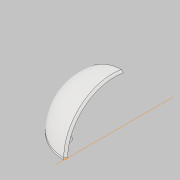
# Autodesk Inventor part: ShellLower
Saved by Autodesk Inventor 2019.2 (Build 232265000, 265)
## iProperties
Created: 2019-01-25
Part Number: ShellLower
Material: ABS-Kunststoff
Document SubType Name: Modeling
Designer: Lion
Density: 1.06 g/cm^3
Appearance: Weiß
Mass: 19.3796 g
Surface Area: 248.39 cm^2
Volume: 18.2826 cm^3
d_inner: 120.000 mm
Author: Lion
## iProperties of the stored document ShellLower_3D-Druck.ipt
Created: 2019-04-11
Part Number: ShellLower_3D-Druck
Material: Generisch
Document SubType Name: Modeling
Designer: Lion
Density: 1 g/cm^3
Appearance: Vorgabe
Author: Lion
Autodesk Inventor part; units mm, degrees
sketch "Skizze1" plane through (0, 0, 0) normal (0, 1, 0) x (-1, 0, 0)
  arc A0 (0, -60) -> (0, 60) centre (0, 0) ccw
  arc A1 (0, -61.5) -> (0, 61.5) centre (0, 0) ccw
  line L0 (0, 60) -> (0, -60) construction
  line L1 (0, 61.5) -> (0, 60)
  line L2 (0, -60) -> (0, -61.5)
  arc A2 (0, 60) -> (0, -60) centre (0, 0) ccw construction
  arc A3 (0, 61.5) -> (0, -61.5) centre (0, 0) ccw construction
  dimension "d_inner" = 120
  dimension "d1" = 123
  constraints: 8 point on circle, 6 end point, 4 centre point, 3 vertical, 2 coincident, 1 midpoint
  measures "d_inner" diameter of A0
  measures "d1" diameter of A1
revolve "Umdrehung1" add sketch "Skizze1" angle 90 about axis through (0, 0, 60) along (0, 0, -1)
sketch "Skizze2" plane through (0, 0, 0) normal (0, -1, 0) x (1, 0, 0)
  arc A0 (0, 60) -> (0, -60) centre (0, 0) ccw projected
  line L0 (0, 60) -> (0, 59)
  line L1 (0, 60) -> (0, -60) construction
  line L2 (-3, 59) -> (-3, 59.925)
  line L3 (0, 59) -> (-3, 59)
  line L4 (0, 0) -> (-60, 0) construction
  dimension "d3" = 1
  dimension "d4" = 3
  constraints: 8 end point, 2 point on circle, 1 horizontal, 1 parallel, 1 perpendicular, 1 point on line
  measures "d3" distance from line of L0.start L3
  measures "d4" distance between parallel lines of L2 L0
sketch "Skizze3" plane through (0, 0, 0) normal (1, 0, 0) x (0, 0, -1)
  line L0 (0, 0) -> (0, 60) construction
  arc A0 (60, 0) -> (-60, 0) centre (0, 0) ccw projected
  line L1 (-60, 0) -> (-59, 0)
  line L2 (-60, 0) -> (60, 0) projected
  line L3 (-59, 0) -> (-59, 2)
  line L4 (-59, 2) -> (-59.9667, 2)
  dimension "d6" = 1
  dimension "d7" = 2
  constraints: 8 end point, 2 point on circle, 2 vertical, 1 perpendicular, 1 point on line
  measures "d6" distance from line of L1.start L3
  measures "d7" distance of L1.end L3.end
ref_plane "Arbeitsebene1" through (0, 0, 0) normal (0, 0, -1) x (-1, 0, 0)
revolve "Umdrehung2" add sketch "Skizze2" angle 180 about axis through (0, 0, 0) along (-1, 0, 0)
revolve "Umdrehung3" add sketch "Skizze3" angle 180 about axis through (0, 0, 0) along (0, -1, 0) contours L4 L3 L1 A0
ref_plane "Arbeitsebene4" through (0, 0, 61) normal (0, 0, -1) x (-1, 0, 0)
chamfer "Fase6" distance 2.5 angle 45 1 edges at (0, 61.5, 0)
sketch "Skizze15" plane through (0, 0, 0) normal (0, -1, 0) x (1, 0, 0)
  line L0 (-2.4995, 61.4492) -> (0, 59) projected
  arc A0 (-2.4995, 61.4492) -> (-2.4995, -61.4492) centre (0, 0) ccw projected
  line L1 (0, -59) -> (-2.4995, -61.4492) projected
  arc A1 (0, 59) -> (0, -59) centre (0, 0) ccw projected
extrude "Extrusion7" add sketch "Skizze15" along normal blind 2.5
chamfer "Fase11" distance 2.5 angle 45 1 edges at (-59, -2.5, 0)
ref_plane "Arbeitsebene21" through (0, 0, 60) normal (0, 1, 0) x (0, 0, -1)
ref_plane "Arbeitsebene20" through (0, 0, 60) normal (1, 0, 0) x (0, 0, -1)
ref_plane "Arbeitsebene25" through (0, 0, 60) normal (0.7071068, 0.7071068, 0) x (0, 0, 1)
ref_plane "Arbeitsebene27" through (-2.4995, -2.5, 61.4492) normal (0, 0, 1) x (1, 0, 0)
ref_plane "Arbeitsebene28" through (-2.4995, -2.5, 2.4492) normal (0, 0, 1) x (1, 0, 0)
ref_plane "Arbeitsebene31" through (-50.9117, 50.9117, 60) normal (0.7071068, -0.7071068, 0) x (0, 0, -1)
ref_plane "Arbeitsebene30" through (-36.7696, 36.7696, 60) normal (0.7071068, -0.7071068, 0) x (0, 0, -1)
ref_plane "Arbeitsebene34" through (-2.4995, 0, -11.4492) normal (0, 0, 1) x (1, 0, 0)
ref_plane "Arbeitsebene33" through (-2.4995, 0, -61.4492) normal (0, 0, 1) x (1, 0, 0)
split "Trennen4" plane through (-2.4995, 0, -11.4492) removes the side toward (0, 0, -1)
ref_plane "Arbeitsebene35" through (0, 0, 60) normal (0.7071068, -0.7071068, 0) x (0, 0, -1)
ref_plane "Arbeitsebene36" through (-10.253, 10.253, 60) normal (0.7071068, -0.7071068, 0) x (0, 0, -1)
ref_plane "Arbeitsebene37" through (-2.4995, -2.5, 52.9492) normal (0, 0, 1) x (1, 0, 0)
sketch "Skizze24" plane through (-2.4995, -2.5, 52.9492) normal (0, 0, 1) x (1, 0, 0)
  line L0 (35.5159, 56.0226) -> (-52.2985, -31.7919) construction
  line L1 (-71.52, 76.5195) -> (16.2944, -11.2949) construction
  line L2 (-7.5768, 7.9801) -> (-12.5265, 12.9298)
  line L3 (-12.5265, 12.9298) -> (-16.0621, 9.3943)
  line L4 (-16.0621, 9.3943) -> (-11.1123, 4.4445)
  line L5 (-11.1123, 4.4445) -> (-7.5768, 7.9801)
  line L6 (-16.0621, 9.3943) -> (-7.5768, 7.9801) construction
  line L7 (-11.1123, 4.4445) -> (-12.5265, 12.9298) construction
  point P0 (2.4995, 2.5)
  point P1 (-11.8194, 8.6872)
  dimension "d150" = 5
  dimension "d151" = 7
  dimension "d152" = 3.25
  constraints: 12 end point, 4 parallel, 1 midpoint, 1 perpendicular, 1 point on line
  measures "d150" distance between parallel lines of L4 L2
  measures "d151" distance between parallel lines of L5 L3
  measures "d152" distance between parallel lines of L2 L1
extrude "Extrusion16" add sketch "Skizze24" along normal up to next
extrude "Extrusion17" add sketch "Skizze24" against normal blind 3.5
fillet "Rundung9" radius 3.5 2 edges at (-11.844, 3.7123, 49.4492) (-16.7938, 8.6621, 49.4492)
mirror "Spiegeln4" about plane through (0, 0, 60) normal (0.7071068, 0.7071068, 0) of "Extrusion16", "Extrusion17", "Rundung9"
sketch "Skizze25" plane through (-10.0763, 5.4801, 52.9492) normal (0.7071068, 0.7071068, 0) x (-0.7071068, 0.7071068, 0)
  line L0 (-30.509, 0) -> (93.6794, 0) construction
  line L1 (3.5, -78.978) -> (3.5, 23.0797) construction
  circle A0 centre (3.5, 0) radius 1.05
  point P0 (-11, -52.9492)
  dimension "d158" = 2.1
  constraints: 2 point on line, 1 centre point
  measures "d158" diameter of A0
extrude "Extrusion18" cut sketch "Skizze25" along normal through all both and the other way through all
ref_plane "Arbeitsebene38" through (-31.1127, 31.1127, 60) normal (0.7071068, -0.7071068, 0) x (0, 0, -1)
ref_plane "Arbeitsebene39" through (-2.4995, -2.5, 29.4492) normal (0, 0, 1) x (1, 0, 0)
sketch "Skizze26" plane through (-31.1127, 31.1127, 60) normal (0.7071068, -0.7071068, 0) x (0, 0, -1)
  line L0 (30.5508, -62.996) -> (30.5508, 61.1923) construction
  line L1 (26.5508, 6.5) -> (34.5508, 6.5)
  line L2 (34.5508, 6.5) -> (34.5508, 0.5)
  line L3 (34.5508, 0.5) -> (26.5508, 0.5)
  line L4 (26.5508, 0.5) -> (26.5508, 6.5)
  line L5 (26.5508, 6.5) -> (34.5508, 0.5) construction
  line L6 (34.5508, 6.5) -> (26.5508, 0.5) construction
  line L7 (-17.0289, 0) -> (92.0289, 0) construction
  point P0 (60, 0)
  point P1 (30.5508, 3.5)
  dimension "d163" = 6
  dimension "d164" = 0.5
  dimension "d165" = 8
  constraints: 12 end point, 2 midpoint, 2 parallel, 1 horizontal, 1 perpendicular, 1 point on line
  measures "d163" distance of L1.end L2.end
  measures "d164" distance between parallel lines of L7 L3
  measures "d165" distance between parallel lines of L4 L2
extrude "Extrusion19" add sketch "Skizze26" against normal up to surface
sketch "Skizze27" plane through (-31.1127, 31.1127, 60) normal (0.7071068, -0.7071068, 0) x (-0.7071068, -0.7071068, 0)
  line L0 (-6.5, 26.5508) -> (-6.5, 34.5508) projected
  line L1 (-0.5, 26.5508) -> (-6.5, 26.5508) projected
  line L2 (-0.5, 34.5508) -> (-0.5, 26.5508) projected
  line L3 (-6.5, 34.5508) -> (-0.5, 34.5508) projected
  point P0 (0, 60)
extrude "Extrusion20" add sketch "Skizze27" along normal blind 4
fillet "Rundung10" radius 4 2 edges at (-25.8094, 30.7591, 25.4492) (-25.8094, 30.7591, 33.4492)
sketch "Skizze28" plane through (-26.5165, 35.7089, 29.4492) normal (0.7071068, 0.7071068, 0) x (-0.7071068, 0.7071068, 0)
  circle A0 centre (0, 0) radius 1.05
  point P0 (-44, -29.4492)
  dimension "d171" = 2.1
  constraints: 1 centre point, 1 coincident
  measures "d171" diameter of A0
extrude "Extrusion21" cut sketch "Skizze28" against normal up to surface (6 mm away)
fillet "Rundung11" [suppressed]
fillet "Rundung12" [suppressed]
fillet "Rundung13" [suppressed]
ref_plane "Arbeitsebene29" through (0, 0, 60) normal (0.7071068, -0.7071068, 0) x (0, 0, -1)
